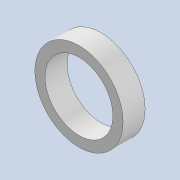
# Autodesk Inventor part: c_roller_1
Saved by Autodesk Inventor 2020 (Build 240168000, 168)
## iProperties
Created: 2021-09-10
Part Number: c_roller_1
Material: Generic
Document SubType Name: Modeling
Designer: Shuang Peng
Density: 1 g/cm^3
Appearance: Default
Author: Shuang Peng
Autodesk Inventor part; units mm, degrees
ref_plane "YZ Plane" through (0, 0, 0) normal (1, 0, 0) x (0, 1, 0)
ref_plane "XZ Plane" through (0, 0, 0) normal (0, 1, 0) x (-1, 0, 0)
ref_plane "XY Plane" through (0, 0, 0) normal (0, 0, 1) x (1, 0, 0)
sketch "Sketch1" plane through (0, 0, 0) normal (0, 0, 1) x (1, 0, 0)
  circle A0 centre (0, 0) radius 3 projected
  circle A1 centre (0, 0) radius 3.075
  circle A2 centre (0, 0) radius 4
  point P0 (0, 0)
  dimension "d0" = 6.15
  dimension "d1" = 8
  constraints: 2 centre point, 2 coincident
  measures "d0" diameter of A1
  measures "d1" diameter of A2
extrude "Extrusion1" add sketch "Sketch1" against normal blind 2 contours A2
ref_plane "Work Plane1" through (0, 0, -1) normal (0, 0, 1) x (1, 0, 0)
sketch "Sketch2" plane through (0, 0, 0) normal (0, 1, 0) x (-1, 0, 0)
  line L0 (4, 0) -> (4, -2) projected
  line L1 (4, -1) -> (3.5, -1)
  line L2 (4, -1) -> (4, -1.5)
  line L3 (4, -1) -> (4, -0.5)
  line L4 (4, -0.5) -> (3.5, -1)
  line L5 (4, -1.5) -> (3.5, -1)
  line L6 (0, 0) -> (0, -2)
  line L7 (-4, -2) -> (4, -2) projected
  dimension "d4" = 0.5
  dimension "d5" = 0.5
  dimension "d6" = 0.5
  constraints: 12 end point, 2 midpoint, 2 point on line, 1 horizontal
  measures "d4" distance of L1.start L1.end
  measures "d5" distance of L1.start L2.end
  measures "d6" distance of L1.start L3.end
revolve "Revolution1" cut sketch "Sketch2" angle 360 about axis through (0, 0, 0) along (0, 0, -1)
fillet "Fillet1" radius 0.2 1 edges at (3.5, 0, -1)
body "Solid1"
